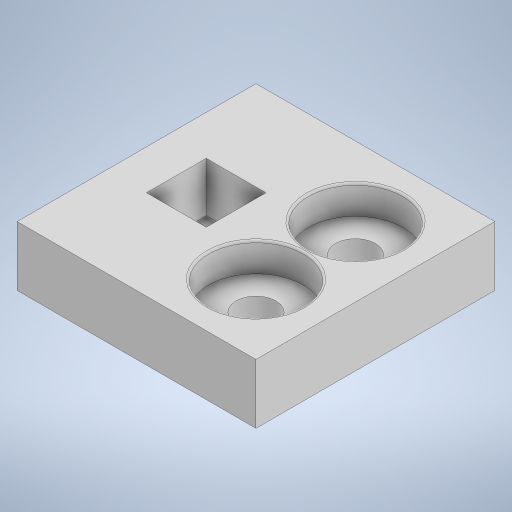
# Autodesk Inventor part: base
Saved by Autodesk Inventor 2024 (Build 280153000, 153)
## iProperties
Created: 2025-01-06
Part Number: base
Material: Generic
Document SubType Name: Modeling
Designer: Pavel
Density: 1 g/cm^3
Appearance: Default
Author: Pavel
Autodesk Inventor part; units mm, degrees
ref_plane "YZ Plane" through (0, 0, 0) normal (1, 0, 0) x (0, 1, 0)
ref_plane "XZ Plane" through (0, 0, 0) normal (0, 1, 0) x (-1, 0, 0)
ref_plane "XY Plane" through (0, 0, 0) normal (0, 0, 1) x (1, 0, 0)
sketch "Sketch1" plane through (0, 0, 0) normal (0, 1, 0) x (-1, 0, 0)
  line L0 (0, 0) -> (11, 0)
  line L1 (0, 0) -> (-13, 0)
  line L2 (-13, 0) -> (-13, 24)
  line L3 (-13, 24) -> (11, 24)
  line L4 (11, 24) -> (11, 0)
  circle A0 centre (-6, 17) radius 2
  circle A1 centre (-6, 7) radius 2
  circle A2 centre (-6, 17) radius 4.65
  circle A3 centre (-6, 7) radius 4.55
  dimension "d0" = 11
  dimension "d1" = 13
  dimension "d2" = 24
  dimension "d3" = 4
  dimension "d4" = 4
  dimension "d5" = 10
  dimension "d12" = 9.3
  dimension "d13" = 9.1
  dimension "d14" = 7
  dimension "d19" = 7
  dimension "d20" = 0
  constraints: 10 end point, 4 centre point, 3 perpendicular, 2 coincident, 2 horizontal
  measures "d0" distance of L0.start L0.end
  measures "d1" distance of L0.start L1.end
  measures "d2" distance of L1.end L2.end
  measures "d3" diameter of A0
  measures "d4" diameter of A1
  measures "d5" distance of A0.centre A1.centre
  measures "d12" diameter of A2
  measures "d13" diameter of A3
  measures "d14" distance from line of L3 A0.centre
  measures "d19" distance from line of L2 A0.centre
  measures "d20" horizontal distance of A0.centre A1.centre
extrude "Extrusion1" add sketch "Sketch1" along normal blind 6 contours L1 L2 L3 L4 L0 | A2 | A3
sketch "Sketch2" plane through (0, 6, 0) normal (0, 1, 0) x (1, 0, 0)
  line L0 (-7, -15) -> (-1, -15)
  line L1 (-1, -15) -> (-1, -9)
  line L2 (-1, -9) -> (-7, -9)
  line L3 (-7, -9) -> (-7, -15)
  line L4 (13, 0) -> (-11, 0) projected
  line L5 (-11, -24) -> (13, -24) projected
  line L6 (-11, 0) -> (-11, -24) projected
  line L7 (-11, -24) -> (-11, 0)
  point P0 (0, 0)
  dimension "d8" = 9
  dimension "d9" = 24
  constraints: 10 end point, 3 equal length, 1 horizontal, 1 perpendicular
  measures "d8" distance between parallel lines of L4 L2
  measures "d9" distance of L4.end L5.start
extrude "Extrusion2" cut sketch "Sketch2" against normal blind 5
sketch "Sketch3" plane through (0, 6, 0) normal (0, 1, 0) x (1, 0, 0)
  circle A0 centre (6, -17) radius 2 projected
  circle A1 centre (6, -17) radius 4.75
  circle A2 centre (6, -7) radius 4.75
  point P0 (0, 0)
  dimension "d15" = 9.5
  dimension "d16" = 9.5
  constraints: 2 centre point, 1 coincident
  measures "d15" diameter of A2
  measures "d16" diameter of A1
extrude "Extrusion3" cut sketch "Sketch3" against normal blind 2.9
fillet "Fillet1" radius 0.2 2 edges at (1.25, 6, 17) (1.25, 6, 7)
body "Solid1"
